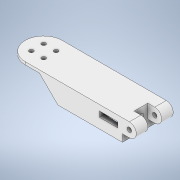
# Autodesk Inventor part: Motor Full Arm
Saved by Autodesk Inventor 2021 (Build 250183000, 183)
## iProperties
Created: 2020-07-16
Part Number: Motor Full Arm
Material: ABS Plastic
Document SubType Name: Modeling
Designer: Andrew
Density: 1.06 g/cm^3
Appearance: Smooth - White
Mass: 43.4154 g
Surface Area: 231.129 cm^2
Volume: 40.9579 cm^3
Author: Andrew
Autodesk Inventor part; units mm, degrees
ref_plane "YZ Plane" through (0, 0, 0) normal (1, 0, 0) x (0, 1, 0)
ref_plane "XZ Plane" through (0, 0, 0) normal (0, 1, 0) x (-1, 0, 0)
ref_plane "XY Plane" through (0, 0, 0) normal (0, 0, 1) x (1, 0, 0)
sketch "Sketch1" plane through (0, 0, 0) normal (0, 1, 0) x (-1, 0, 0)
  line L0 (0, -14) -> (0, 14) projected
ref_plane "Work Plane1" through (0, 3, 0) normal (0, 1, 0) x (1, 0, 0)
sketch "Sketch4" plane through (0, 3, 0) normal (0, 1, 0) x (1, 0, 0)
  circle A0 centre (0, 0) radius 20 projected
  arc A1 (-20, 0) -> (-20, 0) centre (0, 0) ccw
  line L0 (20, 0) -> (20, -125.359)
  line L1 (20, -125.359) -> (-20, -125.359)
  line L2 (-20, -125.359) -> (-20, 0)
  circle A2 centre (0, 0) radius 20
  dimension "d116" = 125.359
  dimension "d117" = 40
  dimension "d118" = 125.359
  dimension "d119" = 40
  dimension "d120" = 40
  constraints: 6 end point, 6 point on circle, 2 coincident, 2 tangent, 1 centre point, 1 concentric, 1 horizontal alignment, 1 parallel, 2 other
  measures "d116" distance of L0.start L0.end
  measures "d117" distance of L0.end L1.end
  measures "d118" distance of L1.end L2.end
  measures "d119" distance from line of A0.start L0
  measures "d120" distance from line of A0.end L0
extrude "Extrusion3" add sketch "Sketch4" against normal blind 3
sketch "Sketch15" plane through (0, 3, 0) normal (0, 1, 0) x (1, 0, 0)
  point P0 (0, 0)
  point P1 (6.7175, 6.7175)
  point P2 (6.7175, -6.7175)
  point P3 (-6.7175, -6.7175)
  point P4 (-6.7175, 6.7175)
  dimension "d99" = 13.435
  dimension "d100" = 13.435
  dimension "d101" = 13.435
  dimension "d102" = 13.435
  dimension "d103" = 6.7175
  dimension "d104" = 6.7175
  dimension "d105" = 0
  dimension "d107" = 6.7175
  measures "d99" distance of point (6.718, -6.718) point (6.718, 6.718)
  measures "d100" distance of point (-6.718, -6.718) point (6.718, -6.718)
  measures "d101" distance of point (-6.718, -6.718) point (-6.718, 6.718)
  measures "d102" distance of point (6.718, 6.718) point (-6.718, 6.718)
  measures "d103" horizontal distance of point (0, 0) point (6.718, 6.718)
  measures "d104" horizontal distance of point (6.718, -6.718) point (0, 0)
  measures "d105" vertical distance of point (-6.718, 6.718) point (6.718, 6.718)
  measures "d107" horizontal distance of point (-6.718, -6.718) point (0, 0)
hole "Hole5" at (6.7175, 3, -6.7175) at (6.7175, 3, 6.7175) at (-6.7175, 3, 6.7175) at (-6.7175, 3, -6.7175) direction (0, -1, 0) diameter 4.5 depth 7.01 tip angle 118 clearance for "Countersunk Flat Head Screw ISO 2009/7046" size "M4" standard "ISO"
sketch "Sketch16" plane through (0, 0, 0) normal (0, -1, 0) x (1, 0, 0)
  line L0 (-20, 0) -> (-20, 125.359) projected
  line L1 (-20, 125.359) -> (20, 125.359)
  line L2 (20, 125.359) -> (20, 15.359)
  line L3 (20, 15.359) -> (-20, 15.359)
  line L4 (-20, 15.359) -> (-20, 125.359)
  line L5 (-15, 15.359) -> (15, 15.359)
  line L6 (15, 15.359) -> (15, 120.359)
  line L7 (15, 120.359) -> (-15, 120.359)
  line L8 (-15, 120.359) -> (-15, 15.359)
  point P0 (0, 0)
  dimension "d121" = 40
  dimension "d122" = 110
  dimension "d123" = 5
  dimension "d124" = 5
  dimension "d125" = 5
  constraints: 16 end point, 4 parallel, 2 horizontal, 2 perpendicular, 1 point on line
  measures "d121" distance of L2.end L3.end
  measures "d122" distance of L1.end L2.end
  measures "d123" distance between parallel lines of L0 L8
  measures "d124" distance between parallel lines of L2 L6
  measures "d125" distance between parallel lines of L1 L7
extrude "Extrusion9" add sketch "Sketch16" along normal blind 20 contours L0 L1 L2 L3 L6 L7 L8
sketch "Sketch17" plane through (-20, 3, 0) normal (-1, 0, 0) x (0, 0, 1)
  line L0 (15.359, -3) -> (35.359, -23)
  line L1 (15.359, -23) -> (120.359, -23) projected
  line L2 (35.359, -23) -> (15.359, -23)
  line L3 (15.359, -3) -> (15.359, -23) projected
  line L4 (15.359, -23) -> (15.359, -3)
  point P0 (0, -3)
  dimension "d128" = 45
  constraints: 6 end point, 2 collinear, 1 point on line
  measures "d128" angle of L3 L0
extrude "Extrusion10" cut sketch "Sketch17" against normal blind 40
ref_plane "Work Plane3" through (15, 0, 57.359) normal (0, 0, -1) x (-1, 0, 0)
ref_plane "Work Plane4" through (15, 0, 57.359) normal (0, 0, -1) x (-1, 0, 0)
ref_plane "Work Plane5" through (15, 0, 37.359) normal (0, 0, -1) x (-1, 0, 0)
sketch "Sketch20" plane through (15, 0, 57.359) normal (0, 0, -1) x (-1, 0, 0)
  point P0 (30, -20)
  point P1 (0, -20)
sketch "Sketch21" plane through (15, 0, 37.359) normal (0, 0, -1) x (-1, 0, 0)
  line L0 (30, -20) -> (15, 0)
  line L1 (15, 0) -> (0, -20)
  line L2 (0, -20) -> (0, 0)
  line L3 (0, 0) -> (30, 0)
  line L4 (30, -20) -> (30, 0)
  line L5 (30, 0) -> (0, 0)
  line L6 (0, 0) -> (0, -20)
  constraints: 14 end point, 1 horizontal
extrude "Rib3" add sketch "Sketch21" along normal mid plane 3 rib yes fills toward (29.95, -10) open curves L4 L0 L1
sketch "Sketch23" plane through (20, 0, 0) normal (1, 0, 0) x (0, 0, -1)
  line L0 (0, 3) -> (-125.359, 3) projected
  line L1 (-125.359, 3) -> (-105.359, 3)
  line L2 (-105.359, 3) -> (-105.359, -20)
  line L3 (-125.359, -20) -> (-35.359, -20) projected
  line L4 (-105.359, -20) -> (-125.359, -20)
  line L5 (-125.359, -20) -> (-125.359, 3)
  line L6 (-35.359, -20) -> (-125.359, -20) projected
  point P0 (0, 0)
  dimension "d167" = 20
  dimension "d168" = 90
  constraints: 8 end point, 2 point on line, 1 perpendicular
  measures "d167" distance from line of L2.end L5
  measures "d168" angle of L3 L2
extrude "Extrusion12" cut sketch "Sketch23" against normal blind 40
ref_plane "Work Plane8" through (-20, -20, 100.359) normal (0, 0, 1) x (1, 0, 0)
ref_plane "Work Plane9" through (-20, -20, 75.359) normal (0, 0, 1) x (1, 0, 0)
sketch "Sketch42" plane through (0, 0, 0) normal (1, 0, 0) x (0, 1, 0)
  line L0 (3, 0) -> (3, 105.359) projected
  line L1 (3, 105.359) -> (3, 120.359)
  line L2 (3, 120.359) -> (-12, 120.359)
  line L3 (-12, 120.359) -> (-12, 105.359)
  line L4 (-20, 105.359) -> (3, 105.359) projected
  circle A0 centre (-4.5, 112.859) radius 2.5
  arc A1 (-4.5, 120.359) -> (-12, 112.859) centre (-4.5, 112.859) ccw
  line L5 (3, 105.359) -> (3, 0) projected
  line L6 (3, 105.359) -> (-12, 105.359)
  arc A2 (3, 112.859) -> (-4.5, 120.359) centre (-4.5, 112.859) ccw
  point P0 (0, 0)
  dimension "d293" = 15
  dimension "d294" = 15
  dimension "d295" = 5
  constraints: 8 end point, 4 point on circle, 3 centre point, 3 midpoint, 3 tangent, 1 coincident, 1 collinear, 1 parallel, 1 perpendicular, 1 point on line, 1 vertical
  measures "d293" distance of L0.end L1.end
  measures "d294" distance of L1.end L2.end
  measures "d295" diameter of A0
extrude "Extrusion20" add sketch "Sketch42" along normal mid plane 40 contours L4 L3 A1 A2 L1
ref_plane "Work Plane10" through (-15, -20, 78.859) normal (1, 0, 0) x (0, 0, -1)
sketch "Sketch44" plane through (-15, -20, 78.859) normal (1, 0, 0) x (0, 0, -1)
  line L0 (-26.5, 0) -> (-21.5, 0)
  line L1 (-21.5, 0) -> (-21.5, 20)
  line L2 (-21.5, 20) -> (-26.5, 20)
  line L3 (-26.5, 20) -> (-26.5, 0)
  line L4 (-26.5, 0) -> (-26.5, 8) projected
  point P0 (78.859, 20)
  point P1 (-26.5, 23)
  dimension "d298" = 5
  constraints: 8 end point, 2 parallel, 1 collinear, 1 horizontal, 1 perpendicular
  measures "d298" distance of L2.end L1.end
extrude "Extrusion21" add sketch "Sketch44" along normal blind 30
sketch "Sketch45" plane through (-20, 0, 0) normal (-1, 0, 0) x (0, 0, 1)
  line L0 (80.359, -3) -> (100.359, -3)
  line L1 (100.359, -3) -> (100.359, -9)
  line L2 (100.359, -9) -> (80.359, -9)
  line L3 (80.359, -9) -> (80.359, -3)
  line L4 (0, 3) -> (105.359, 3) projected
  point P0 (0, 0)
  dimension "d301" = 6
  dimension "d302" = 6
  dimension "d305" = 20
  constraints: 8 end point, 2 parallel, 1 horizontal, 1 perpendicular
  measures "d301" distance of L0.end L1.end
  measures "d302" distance between parallel lines of L4 L0
  measures "d305" distance of L0.start L0.end
extrude "Extrusion22" cut sketch "Sketch45" against normal blind 40
sketch "Sketch46" plane through (0, 3, 0) normal (0, 1, 0) x (1, 0, 0)
  line L0 (-7.5, -105.359) -> (7.5, -105.359)
  line L1 (7.5, -105.359) -> (7.5, -120.359)
  line L2 (7.5, -120.359) -> (-7.5, -120.359)
  line L3 (-7.5, -120.359) -> (-7.5, -105.359)
  line L4 (20, -105.359) -> (-20, -105.359) projected
  line L5 (-20, 0) -> (-20, -112.859) projected
  point P0 (0, 0)
  dimension "d306" = 15
  dimension "d307" = 0
  dimension "d308" = 15
  dimension "d309" = 12.5
  constraints: 8 end point, 2 parallel, 1 horizontal, 1 perpendicular
  measures "d306" distance of L0.end L1.end
  measures "d307" distance between parallel lines of L4 L0
  measures "d308" distance of L1.end L2.end
  measures "d309" distance between parallel lines of L5 L3
extrude "Extrusion23" cut sketch "Sketch46" against normal blind 40
sketch "Sketch39" plane through (15, 0, 35.859) normal (0, 0, -1) x (-1, 0, 0)
  line L0 (15, 0) -> (30, 0) projected
  line L1 (30, 0) -> (30, -20) projected
  point P0 (27.5, -12)
  dimension "d282" = 12
  dimension "d283" = 2.5
  measures "d282" distance from line of L0 point (27.5, -12)
  measures "d283" distance from line of L1 point (27.5, -12)
hole "Hole14" at (-12.5, -12, 35.859) direction (0, 0, 1) diameter 3 depth 40 tip angle 118
sketch "Sketch48" plane through (-20, -20, 105.359) normal (0, 0, 1) x (1, 0, 0)
  circle A0 centre (20, 14) radius 3.1
  line L0 (12.5, 23) -> (12.5, 8) projected
  line L1 (12.5, 23) -> (27.5, 23) projected
  point P0 (20, 20)
  dimension "d331" = 6.2
  dimension "d332" = 7.5
  dimension "d333" = 9
  constraints: 1 centre point
  measures "d331" diameter of A0
  measures "d332" distance from line of L0 A0.centre
  measures "d333" distance from line of L1 A0.centre
extrude "Extrusion26" cut sketch "Sketch48" against normal blind 5
sketch "Sketch49" plane through (15, 0, 57.359) normal (0, 0, -1) x (-1, 0, 0)
  line L0 (0, -20) -> (30, -20)
  line L1 (30, -20) -> (30, 0)
  line L2 (30, 0) -> (0, 0)
  line L3 (0, 0) -> (0, -20)
  point P0 (15, 0)
  constraints: 8 end point, 2 parallel, 1 horizontal, 1 perpendicular
extrude "Extrusion27" add sketch "Sketch49" along normal blind 3
sketch "Sketch50" plane through (15, 0, 57.359) normal (0, 0, 1) x (1, 0, 0)
  circle A0 centre (-25, -5.498) radius 3
  circle A1 centre (-25, -5.498) radius 4
  circle A2 centre (-5, -5.498) radius 3
  circle A3 centre (-5, -5.498) radius 4
  line L0 (0, 0) -> (0, -20) projected
  line L1 (-30, -20) -> (-30, 0) projected
  line L2 (0, -20) -> (-30, -20) projected
  point P0 (-15, 0)
  dimension "d338" = 6
  dimension "d339" = 8
  dimension "d340" = 6
  dimension "d341" = 8
  dimension "d342" = 5
  dimension "d343" = 5
  dimension "d344" = 14.502
  dimension "d345" = 14.502
  constraints: 4 centre point, 2 coincident
  measures "d338" diameter of A0
  measures "d339" diameter of A1
  measures "d340" diameter of A2
  measures "d341" diameter of A3
  measures "d342" distance from line of L0 A2.centre
  measures "d343" distance from line of L1 A0.centre
  measures "d344" distance from line of L2 A2.centre
  measures "d345" distance from line of L2 A0.centre
extrude "Extrusion28" add sketch "Sketch50" along normal blind 3
sketch "Sketch51" plane through (-20, -20, 75.359) normal (0, 0, 1) x (1, 0, 0)
  line L0 (35, 20) -> (5, 20)
  line L1 (5, 20) -> (5, 0)
  line L2 (5, 0) -> (35, 0)
  line L3 (35, 0) -> (35, 20)
  circle A0 centre (30, 14.502) radius 3
  circle A1 centre (10, 14.502) radius 3
  point P0 (20, 20)
  dimension "d348" = 6
  dimension "d349" = 6
  dimension "d350" = 5
  dimension "d351" = 5
  dimension "d352" = 14.502
  dimension "d353" = 14.502
  constraints: 8 end point, 2 centre point, 2 parallel, 1 horizontal, 1 perpendicular
  measures "d348" diameter of A0
  measures "d349" diameter of A1
  measures "d350" distance from line of L3 A0.centre
  measures "d351" distance from line of L1 A1.centre
  measures "d352" distance from line of L2 A0.centre
  measures "d353" vertical distance of L1.end A1.centre
extrude "Extrusion29" add sketch "Sketch51" along normal blind 3
body "Solid1"
